Autodesk Fusion 360 part; units mm, degrees
(part 7 of 7)
  spline S20 degree 5 poles (9.3559, -0.8768) (9.3606, -0.8772) (9.3699, -0.878) (9.3839, -0.8787) (9.4026, -0.879) (9.426, -0.8784) (9.4495, -0.8772) (9.473, -0.8755) (9.4965, -0.8735) (9.52, -0.8714) (9.5435, -0.8691) (9.567, -0.8666) (9.5906, -0.8638) (9.6142, -0.8607) (9.6377, -0.8572) (9.6613, -0.8534) (9.6849, -0.8494) (9.7085, -0.8451) (9.7321, -0.8406) (9.7557, -0.836) (9.7793, -0.8311) (9.8029, -0.8261) (9.8265, -0.8208) (9.8501, -0.8153) (9.8737, -0.8096) (9.8973, -0.8037) (9.9209, -0.7977) (9.9445, -0.7914) (9.968, -0.7849) (9.9916, -0.7783) (10.0152, -0.7715) (10.0388, -0.7645) (10.0623, -0.7574) (10.0859, -0.7501) (10.1095, -0.7426) (10.133, -0.7349) (10.1565, -0.7271) (10.1801, -0.7191) (10.2036, -0.711) (10.2271, -0.7027) (10.2506, -0.6942) (10.2741, -0.6856) (10.2976, -0.6768) (10.321, -0.6679) (10.3445, -0.6588) (10.3679, -0.6496) (10.3913, -0.6402) (10.4148, -0.6307) (10.4382, -0.621) (10.4615, -0.6112) (10.4849, -0.6013) (10.5083, -0.5912) (10.5316, -0.5809) (10.5549, -0.5705) (10.5782, -0.56) (10.6015, -0.5493) (10.6248, -0.5385) (10.6481, -0.5276) (10.6713, -0.5165) (10.6945, -0.5053) (10.7177, -0.4939) (10.7409, -0.4824) (10.7641, -0.4708) (10.7872, -0.4591) (10.8103, -0.4472) (10.8334, -0.4352) (10.8565, -0.423) (10.8796, -0.4107) (10.9026, -0.3983) (10.9256, -0.3858) (10.9486, -0.3731) (10.967, -0.3629) (10.9807, -0.3552) (10.9899, -0.35) (10.9945, -0.3474) knots 0 0 0 0 0 0 0.01428571 0.02857143 0.04285714 0.05714286 0.07142857 0.08571429 0.1 0.11428571 0.12857143 0.14285714 0.15714286 0.17142857 0.18571429 0.2 0.21428571 0.22857143 0.24285714 0.25714286 0.27142857 0.28571429 0.3 0.31428571 0.32857143 0.34285714 0.35714286 0.37142857 0.38571429 0.4 0.41428571 0.42857143 0.44285714 0.45714286 0.47142857 0.48571429 0.5 0.51428571 0.52857143 0.54285714 0.55714286 0.57142857 0.58571429 0.6 0.61428571 0.62857143 0.64285714 0.65714286 0.67142857 0.68571429 0.7 0.71428571 0.72857143 0.74285714 0.75714286 0.77142857 0.78571429 0.8 0.81428571 0.82857143 0.84285714 0.85714286 0.87142857 0.88571429 0.9 0.91428571 0.92857143 0.94285714 0.95714286 0.97142857 0.98571429 1 1 1 1 1 1
  arc A47 (10.9945, -0.3474) -> (10.9945, 0.3474) centre (0, 0) ccw
  spline S21 degree 5 poles (10.9945, 0.3474) (10.9899, 0.35) (10.9807, 0.3552) (10.967, 0.3629) (10.9486, 0.3731) (10.9256, 0.3858) (10.9026, 0.3983) (10.8796, 0.4107) (10.8565, 0.423) (10.8334, 0.4352) (10.8103, 0.4472) (10.7872, 0.4591) (10.7641, 0.4708) (10.7409, 0.4824) (10.7177, 0.4939) (10.6945, 0.5053) (10.6713, 0.5165) (10.6481, 0.5276) (10.6248, 0.5385) (10.6015, 0.5493) (10.5782, 0.56) (10.5549, 0.5705) (10.5316, 0.5809) (10.5083, 0.5912) (10.4849, 0.6013) (10.4615, 0.6112) (10.4382, 0.621) (10.4148, 0.6307) (10.3913, 0.6402) (10.3679, 0.6496) (10.3445, 0.6588) (10.321, 0.6679) (10.2976, 0.6768) (10.2741, 0.6856) (10.2506, 0.6942) (10.2271, 0.7027) (10.2036, 0.711) (10.1801, 0.7191) (10.1565, 0.7271) (10.133, 0.7349) (10.1095, 0.7426) (10.0859, 0.7501) (10.0623, 0.7574) (10.0388, 0.7645) (10.0152, 0.7715) (9.9916, 0.7783) (9.968, 0.7849) (9.9445, 0.7914) (9.9209, 0.7977) (9.8973, 0.8037) (9.8737, 0.8096) (9.8501, 0.8153) (9.8265, 0.8208) (9.8029, 0.8261) (9.7793, 0.8311) (9.7557, 0.836) (9.7321, 0.8406) (9.7085, 0.8451) (9.6849, 0.8494) (9.6613, 0.8534) (9.6377, 0.8572) (9.6142, 0.8607) (9.5906, 0.8638) (9.567, 0.8666) (9.5435, 0.8691) (9.52, 0.8714) (9.4965, 0.8735) (9.473, 0.8755) (9.4495, 0.8772) (9.426, 0.8784) (9.4026, 0.879) (9.3839, 0.8787) (9.3699, 0.878) (9.3606, 0.8772) (9.3559, 0.8768) knots -1 -1 -1 -1 -1 -1 -0.98571429 -0.97142857 -0.95714286 -0.94285714 -0.92857143 -0.91428571 -0.9 -0.88571429 -0.87142857 -0.85714286 -0.84285714 -0.82857143 -0.81428571 -0.8 -0.78571429 -0.77142857 -0.75714286 -0.74285714 -0.72857143 -0.71428571 -0.7 -0.68571429 -0.67142857 -0.65714286 -0.64285714 -0.62857143 -0.61428571 -0.6 -0.58571429 -0.57142857 -0.55714286 -0.54285714 -0.52857143 -0.51428571 -0.5 -0.48571429 -0.47142857 -0.45714286 -0.44285714 -0.42857143 -0.41428571 -0.4 -0.38571429 -0.37142857 -0.35714286 -0.34285714 -0.32857143 -0.31428571 -0.3 -0.28571429 -0.27142857 -0.25714286 -0.24285714 -0.22857143 -0.21428571 -0.2 -0.18571429 -0.17142857 -0.15714286 -0.14285714 -0.12857143 -0.11428571 -0.1 -0.08571429 -0.07142857 -0.05714286 -0.04285714 -0.02857143 -0.01428571 0 0 0 0 0 0
  line L30 (9.3559, 0.8768) -> (9.279, 0.8697)
  arc A48 (8.642, 1.3652) -> (9.279, 0.8697) centre (9.2248, 1.4572) ccw
  circle A49 centre (0, 0) radius 4
  line L31 (0, 0) -> (-2.8, 0)
  line L32 (-2.8, 0) -> (-2.8, 9.5032)
  line L33 (-2.8, 9.5032) -> (0, 9.5032)
  line L34 (0, 9.5032) -> (0, 0)
  line L35 (0, 0) -> (2.8, 0)
  line L36 (2.8, 0) -> (2.8, 9.5032)
  line L37 (2.8, 9.5032) -> (0, 9.5032)
  line L38 (0, 9.5032) -> (0, 0)
  dimension "d18" = 2.8
  dimension "d19" = 2.8
  constraint horizontal L31
  constraint vertical L32
  constraint horizontal L33
  constraint vertical L34
  constraint coincident A1.centre A2.centre
  constraint horizontal L35
  constraint vertical L36
  constraint horizontal L37
  constraint vertical L38
  measures "d18" distance of A1.centre L31.end
  measures "d19" distance of A1.centre L35.end
extrude "Extrude3'" add sketch "Sketch3 (2)" along normal blind 5 separate body contours L0 A0 L1 L2 L3 L5 A2 L6 L7 A3 A4 A5 L8 A6 L9 S0 A7 S1 L10 A8 A9 A10 L11 S2 A11 S3 L12 A12 A13 A14 L13 S4 A15 S5 L14 A16 A17 A18 L15 S6 A19 S7 L16 A20 A21 A22 L17 S8 A23 S9 L18 A24 A25 A26 L19 S10 A27 S11 L20 A28 A29 A30 L21 S12 A31 S13 L22 A32 A33 A34 L23 S14 A35 S15 L24 A36 A37 A38 L25 S16 A39 S17 L26 A40 A41 A42 L27 S18 A43 S19 L28 A44 A45 A46 L29 S20 A47 S21 L30 A48 A49 L32 L36 makes body 2
extrude "Extrude6" cut sketch "Sketch3 (2)" against normal blind 2.5 contours L3 A1 L4 A49 L34 L36 L38 | L3 A1 L4 L34 L36 L37 L38 | L4 L5 A49 L32 L34 L38 | L4 L5 L32 L33 L34 L38 bodies 1 in component "Spur Gear (20 teeth)"
component "Spur Gear (20 teeth)" placed x (1, 0, 0) y (0, 1, 0) z (0, 0, 1) at (0, 0, 0)

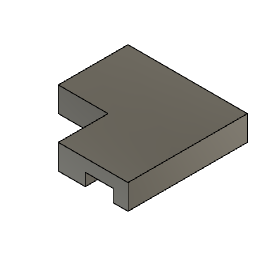
design "corner"
Autodesk Fusion 360 part; units mm, degrees
sketch "Sketch1" plane through (0, 0, 0) normal (0, 0, 1) x (1, 0, 0)
  circle A0 centre (0, 0) radius 22
  circle A1 centre (0, 0) radius 11
  line L0 (0, 0) -> (0, 20)
  line L1 (0, 0) -> (26, 0)
  line L2 (0, 0) -> (28, 0)
  line L3 (28, 0) -> (28, 28)
  line L4 (28, 28) -> (0, 28)
  line L5 (0, 28) -> (0, 0)
  line L6 (0, 11) -> (0, 22) construction
  line L7 (11, 0) -> (13, 0) construction
  arc A2 (11, 0) -> (0, 11) centre (0.4983, 0.4983) ccw construction
  dimension "d1" = 44
  dimension "d2" = 22
  constraint coincident A0.centre A1.centre
  constraint concentric A0 A1
  constraint vertical L0
  constraint perpendicular L0 L1
  constraint horizontal L2
  constraint vertical L3
  constraint horizontal L4
  constraint vertical L5
  constraint coincident A1 L6.start
  constraint coincident L0 L6.start
  constraint coincident L0 L6.end
  constraint coincident A0 L6.end
  constraint coincident A1 L7.start
  constraint coincident L1 L7.start
  constraint midpoint L1 L7.end
  constraint perpendicular L6 L7
  measures "d1" diameter of A0
  measures "d2" diameter of A1
extrude "Extrude1" add sketch "Sketch1" along normal blind 10 contours A0 A1 L0 L1 L2 L5 | A0 L1 L2 L3 L4 L5 | A1 L0 L1 L2 L5 picked at (3.0991, 17.2211) picked at (3.5055, 6.4199)
extrude "Extrude2" cut sketch "Sketch1" along normal blind 5 contours A0 A1 L0 L1 L2 L5 picked at (3.0991, 17.2211)
extrude "Extrude4" add 1 faces at (0, 3.6667, 5) along direction (-1, 0, 0) blind 20
sketch "Sketch5" plane through (0, 0, 0) normal (0, 1, 0) x (1, 0, 0)
  line L0 (28, 0) -> (0, 0)
  line L1 (0, 0) -> (0, -10)
  line L2 (0, -10) -> (28, -10)
  line L3 (28, -10) -> (28, 0)
  line L4 (22, -5) -> (10.8427, -5)
  line L5 (10.8427, -5) -> (10.8427, 0)
  line L6 (10.8427, 0) -> (22, 0)
  line L7 (22, 0) -> (22, -5)
  constraint horizontal L0
  constraint vertical L1
  constraint horizontal L2
  constraint vertical L3
  constraint horizontal L4
  constraint vertical L5
  constraint horizontal L6
  constraint vertical L7
  constraint coincident L0 L5.end
extrude "Extrude5" add sketch "Sketch5" against normal blind 20 contours L0 L1 L2 L3 L4 L5 L7
sketch "Sketch6" plane through (0, 0, 0) normal (0, 0, -1) x (1, 0, 0)
  arc A0 (0, -11) -> (11, 0) centre (0, 0) ccw
  line L0 (11, 0) -> (10.8427, 0)
  line L1 (10.8427, 0) -> (10.8427, 20)
  line L2 (10.8427, 20) -> (0, 20)
  line L3 (0, 20) -> (0, 0)
  line L4 (0, 0) -> (-20, 0)
  line L5 (-20, 0) -> (-20, -11)
  line L6 (-20, -11) -> (0, -11)
  line L7 (10.8427, 0) -> (0, 0)
  line L8 (0, 0) -> (0, -11)
  circle A1 centre (0, 0) radius 5
  dimension "d18" = 10
  constraint coincident L0.end L1.start
  constraint coincident A0.centre L3.end
  constraint coincident A0.start L6.end
  measures "d18" diameter of A1
extrude "Extrude6" cut sketch "Sketch6" against normal blind 5 contours A0 L0 L7 L8 A1
fillet "Fillet1" radius 5 2 edges at (10.8427, 0, 2.5) (0, 11, 2.5)

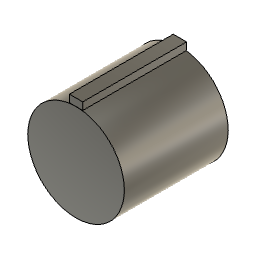
design "thruster"
Autodesk Fusion 360 part; units mm, degrees
sketch "Sketch1" plane through (0, 0, 0) normal (0, 1, 0) x (1, 0, 0)
  circle A0 centre (0, 0) radius 32.5
  dimension "d1" = 65
  constraint coincident A0.centre origin
  measures "d1" diameter of A0
extrude "Extrude1" add sketch "Sketch1" along normal blind 70 makes body 1
sketch "Sketch2" plane through (0, 0, 0) normal (0, 1, 0) x (1, 0, 0)
  line L0 (0, 0) -> (0, -32.5) construction
  line L1 (0, -32.5) -> (-4.5, -32.5)
  line L2 (-4.5, -32.5) -> (-4.5, -37.5)
  line L3 (-4.5, -37.5) -> (0, -37.5)
  line L4 (0, -37.5) -> (0, -32.5)
  line L5 (0, -32.5) -> (4.5, -32.5)
  line L6 (4.5, -32.5) -> (4.5, -37.5)
  line L7 (4.5, -37.5) -> (0, -37.5)
  line L8 (0, -37.5) -> (0, -32.5)
  dimension "d4" = 32.5
  dimension "d5" = 4.5
  dimension "d6" = 5
  dimension "d7" = 5
  constraint coincident L0.start origin
  constraint vertical L0
  constraint horizontal L1
  constraint vertical L2
  constraint horizontal L3
  constraint vertical L4
  constraint horizontal L5
  constraint vertical L6
  constraint horizontal L7
  constraint vertical L8
  measures "d4" distance of L0.start L0.end
  measures "d5" distance of L0.end L1.end
  measures "d6" distance of L0.end L3.end
  measures "d7" distance of L0.end L3.end
extrude "Extrude2" add sketch "Sketch2" along normal blind 70 separate body makes body 2
